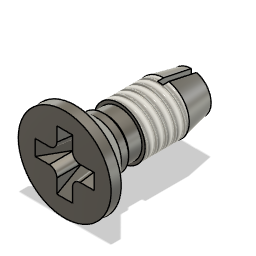
final_combined_updated (Autodesk Fusion 360 archive; units mm, degrees)
design "Type I Cross Recessed Flat Countersunk Head Tapping Screw ASME B18.6.5M M2.5x0.45 x 6 Type D Steel Grade 2 Plain"
description: Type I Cross Recessed Flat Countersunk Head Tapping Screw ASME B18.6.5M M2.5x0.45 x 6 Type D
part number: CRFCHTS ASME B18.6.5M - M2.5x0.45 x 6 - D - I Steel Grade 2 Plain
Autodesk Fusion 360 part; units mm, degrees
sketch "Sketch1" plane through (0, 0, 0) normal (0, 1, 0) x (1, 0, 0)
  line L0 (0, -2.68) -> (-2.2, -2.68)
  line L1 (-2.2, -2.68) -> (-2.2, -2.2)
  line L2 (-2.2, -2.2) -> (-1.18, -1.18)
  line L3 (-1.18, -1.18) -> (0, 0) construction
  line L4 (-1.25, 3.32) -> (0, 3.32)
  line L5 (0, 3.32) -> (0, -2.68)
  line L6 (-1.18, -1.18) -> (-1.18, -0.83)
  line L7 (-1.18, -0.83) -> (-1.0625, -0.7125)
  line L8 (-1.0625, -0.7125) -> (-1.0625, -0.08)
  line L9 (-1.0625, -0.08) -> (-1.25, -0.08)
  line L10 (-1.25, -0.08) -> (-1.25, 3.32)
  line L11 (-1.18, -1.18) -> (0, -1.18) construction
  dimension "d5" = 45
  dimension "d9" = 2.5
  dimension "d11" = 4.4
  dimension "d68" = 1.5
  dimension "d94" = 3.4
  dimension "d95" = 2.125
  dimension "d96" = 45
  dimension "d97" = 2.36
  dimension "d102" = 6
  dimension "d103" = 0.35
  constraint perpendicular L0 L1
  constraint collinear L2 L3
  constraint perpendicular L0 L5
  constraint collinear L3.end L0.start L4.end
  constraint coincident L3.end L5
  constraint coincident origin L3
  constraint horizontal L0
  constraint vertical L6
  constraint parallel L6 L8
  constraint perpendicular L8 L9
  constraint perpendicular L4 L10
  constraint vertical L10
  constraint coincident L5 L11.end
  constraint perpendicular L5 L11
  measures "d5" angle of L3 L5
  measures "d68" distance of L0 L2.end
  measures "d94" distance of L4 L9
  measures "d96" angle of L6 L7
  measures "d102" distance of L0.start L4
  measures "d103" distance of L6.end L11
revolve "Revolve1" add sketch "Sketch1" angle 360 about axis through (0, 0, -3.32) along (0, 0, 1) makes body 1
sketch "Sketch2" plane through (0, 0, 2.68) normal (0, 0, 1) x (1, 0, 0)
  line L0 (-0.37, 0.37) -> (-1.4, 0.37)
  line L1 (-1.4, 0.37) -> (-1.4, -0.37)
  line L2 (-1.4, -0.37) -> (-0.37, -0.37)
  line L3 (-0.37, -0.37) -> (-0.37, -1.4)
  line L4 (-0.37, -1.4) -> (0.37, -1.4)
  line L5 (0.37, -1.4) -> (0.37, -0.37)
  line L6 (0.37, -0.37) -> (1.4, -0.37)
  line L7 (1.4, -0.37) -> (1.4, 0.37)
  line L8 (1.4, 0.37) -> (0.37, 0.37)
  line L9 (0.37, 0.37) -> (0.37, 1.4)
  line L10 (0.37, 1.4) -> (-0.37, 1.4)
  line L11 (-0.37, 1.4) -> (-0.37, 0.37)
  dimension "d104" = 0.74
  dimension "d106" = 360
  dimension "d107" = 2.8
  constraint horizontal L0
  constraint perpendicular L0 L1
  constraint horizontal L2
  constraint vertical L0.start L2.end
  constraint coincident L0.start L11.end
  measures "d104" distance of L0 L1.end
  measures "d107" distance of L3.end L10
extrude "Extrude1" add sketch "Sketch2" against normal blind 1.78 draft -4 separate body makes body 2
draft "Draft1" angle -30 neutral plane through (0, 0, 2.68) pull (0, 0, 1) 4 faces at (1.3585, 0.0818, 2.0867) (-0.0818, 1.3585, 2.0867) (-0.0818, -1.3585, 2.0867) (-1.3585, 0.0818, 2.0867) on bodies 2
fillet "Fillet3" radius 0.364 4 edges at (0.3078, 0.3078, 1.79) (-0.3078, 0.3078, 1.79) (-0.3078, -0.3078, 1.79) (0.3078, -0.3078, 1.79) on bodies 2
combine "Combine1" operation cut target body 1 tool bodies 2
thread "Thread1" "ANSI Metric M Profile 2.5 M2.5x0.45 6g" major diameter 2.43 minor diameter 1.9165 pitch 0.45 angle 60 resizes the face on face at (-1.2484, 0.0623, -1.0533) on bodies 1
sketch "Sketch5" plane through (0, 0, 0) normal (0, 1, 0) x (1, 0, 0)
  line L0 (-1.275, 3.32) -> (-1.275, 1.72)
  line L1 (-1.275, 1.72) -> (-0.94, 3.32)
  line L2 (0, 3.32) -> (0, -2.68)
  line L3 (0, 3.32) -> (-1.275, 3.32)
  dimension "d81" = 1.275
  dimension "d110" = 0.94
  dimension "d111" = 1.6
  constraint vertical L0
  constraint coincident L2.start L3.start
  constraint perpendicular L0 L3
  constraint coincident L1.end L3
  measures "d81" distance of origin L0
  measures "d110" distance of L1.end L2
  measures "d111" distance of L0.end L3
revolve "Revolve2" cut sketch "Sketch5" angle 360 about axis through (0, 0, -3.32) along (0, 0, 1) bodies 1
sketch "Sketch6" plane through (0, 0, -3.32) normal (0, 0, -1) x (-1, 0, 0)
  line L0 (-0.25, 2.2) -> (0, 2.2)
  line L1 (0, 2.2) -> (0, 0)
  line L2 (0, 0) -> (-0.25, 0)
  circle A0 centre (0, 0) radius 0.94
  line L3 (-0.25, 2.2) -> (-0.25, 0)
  dimension "d112" = 0.25
  dimension "d113" = 2.2
  constraint horizontal L2
  constraint coincident L1.end L2.start
  constraint perpendicular L1 L2
  constraint perpendicular L0 L1
  constraint perpendicular L0 L3
  measures "d112" distance of L0.end L3
  measures "d113" distance of L1.end L0
extrude "Extrude2" cut sketch "Sketch6" against normal blind 1.6 contours L0 L1 A0 L3 | L1 L2 A0 L3 picked at (-0.1667, 0.302) bodies 1
equation "d5 = adsk_headang * 0.5"
equation "d9 = adsk_nomdia"
equation "d11 = adsk_headdia"
equation "adsk_nomlen = 6.00 mm"
equation "adsk_headh = 1.50 mm"
equation "adsk_headdia = 4.40 mm"
equation "adsk_nomdia = 2.50 mm"
equation "adsk_headang = 90.00 deg"
equation "adsk_phildia = 2.80 mm"
equation "d31 = -adsk_phildepth"
equation "adsk_philwidth = 0.74 mm"
equation "adsk_phildepth = 1.78 mm"
equation "adsk_startlen = 1.60 mm"
equation "d68 = adsk_headh"
equation "d73 = -adsk_startlen"
equation "adsk_endpointdia = 1.88 mm"
equation "d81 = adsk_nomdia * 0.51"
equation "d86 = ( adsk_nomdia * 0.5 ) * tan(90 deg - adsk_headang * 0.5) + adsk_headh"
equation "adsk_thrlen = 3.40 mm"
equation "adsk_grpdia = 2.36 mm"
equation "adsk_grplen = 0.35 mm"
equation "adsk_shlang = 45.00 deg"
equation "d94 = adsk_thrlen"
equation "d95 = adsk_shnkdia"
equation "d96 = adsk_shlang"
equation "d97 = adsk_grpdia"
equation "adsk_shnkdia = adsk_nomdia * 0.85"
equation "d102 = adsk_nomlen"
equation "d103 = adsk_grplen"
equation "d104 = adsk_philwidth"
equation "d107 = adsk_phildia"
equation "d109 = adsk_phildia * 0.13"
equation "d110 = adsk_endpointdia / 2"
equation "d111 = adsk_startlen"
equation "d112 = adsk_nomdia / 10"
equation "d113 = adsk_headdia / 2"

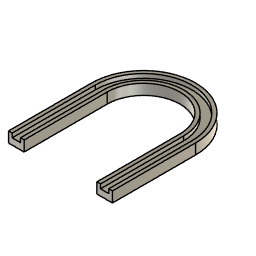
design "supporter"
Autodesk Fusion 360 part; units mm, degrees
sketch "Sketch1" plane through (0, 0, 0) normal (0, 0, 1) x (1, 0, 0)
  line L0 (-65, 0) -> (67.0686, 0)
  line L1 (-35, 0) -> (-35, -80)
  line L2 (-50, 0) -> (-50, -80)
  line L3 (35, 0) -> (35, -80)
  line L4 (50, 0) -> (50, -80)
  line L5 (35, -80) -> (50, -80)
  line L6 (-50, -80) -> (-35, -80)
  arc A0 (35, 0) -> (-35, 0) centre (0, 0) ccw
  arc A1 (50, 0) -> (-50, 0) centre (0, 0) ccw
  arc A2 (38.5, 0) -> (-38.5, 0) centre (0, 0) ccw
  arc A3 (46.5, 0) -> (-46.5, 0) centre (0, 0) ccw
  line L7 (-38.5, 0) -> (-38.5, -80)
  line L8 (-46.5, 0) -> (-46.5, -80)
  line L9 (38.5, 0) -> (38.5, -80)
  line L10 (46.5, 0) -> (46.5, -80)
  dimension "d1" = 70
  dimension "d2" = 100
  dimension "d3" = 80
  dimension "d4" = 80
  dimension "d5" = 80
  dimension "d8" = 77
  dimension "d9" = 93
  constraint coincident A0.centre A1.centre
  constraint horizontal L0
  constraint coincident L0 L1.start
  constraint tangent L1 A0
  constraint perpendicular L0 L1
  constraint coincident L0 L2.start
  constraint tangent L2 A1
  constraint coincident L0 L3.start
  constraint tangent L3 A0
  constraint coincident L0 L4.start
  constraint tangent L4 A1
  constraint perpendicular L4 L5
  constraint concentric A0 A3
  constraint coincident L0 A2.end
  constraint coincident L0 A2.start
  constraint coincident L0 A3.end
  constraint coincident L0 A3.start
  constraint coincident L6 L7.end
  constraint tangent A2 L7
  constraint coincident L6 L8.end
  constraint tangent A3 L8
  constraint coincident L5 L9.end
  constraint tangent A2 L9
  constraint coincident L5 L10.end
  constraint tangent A3 L10
  measures "d1" diameter of A0
  measures "d2" diameter of A1
  measures "d3" distance of L1.start L1.end
  measures "d4" distance of L2.start L2.end
  measures "d5" distance of L4.start L4.end
  measures "d8" diameter of A2
  measures "d9" diameter of A3
extrude "Extrude2" add sketch "Sketch1" along normal blind 6 contours L0 A1 A3 | L0 L2 L6 L8 | L0 L4 L5 L10 | L0 A0 A2 | L0 L1 L6 L7 | L0 L3 L5 L9 makes body 1 at (36.1667, -53.3333, 0) makes body 2 at (-47.6667, -53.3333, 0)
extrude "Extrude3" add sketch "Sketch1" along normal blind 2 separate body contours L0 A2 A3 | L0 L6 L7 L8 | L0 L5 L9 L10 makes body 3
extrude "Extrude4" add sketch "Sketch1" against normal blind 4.1 contours L0 A1 A3 | L0 L2 L6 L8 | L0 A2 A3 | L0 L6 L7 L8 | L0 L4 L5 L10 | L0 A0 A2 | L0 L1 L6 L7 | L0 L5 L9 L10 | L0 L3 L5 L9 bodies 1 2 3

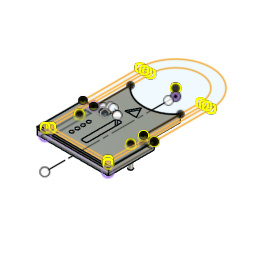
design "cap"
Autodesk Fusion 360 part; units mm, degrees
ref_plane "WorkPlane1" through (0, 0, 100) normal (0, 0, 1) x (1, 0, 0)
sketch "Sketch3" plane through (0, 0, 100) normal (0, 0, 1) x (1, 0, 0)
  line L0 (50, -80) -> (50, 0)
  arc A0 (50, 0) -> (-50, 0) centre (0, 0) ccw
  arc A1 (35, 0) -> (-35, 0) centre (0, 0) ccw
  line L1 (35, 0) -> (35, -80)
  line L2 (35, -80) -> (50, -80)
  line L3 (-50, 0) -> (-50, -80)
  line L4 (-50, -80) -> (-35, -80)
  line L5 (-35, -80) -> (-35, 0)
  circle A2 centre (-36, -99) radius 3
  circle A3 centre (36, -99) radius 3
  line L6 (40, -135) -> (-40, -135)
  line L7 (-40, -135) -> (-40, 0)
  line L8 (40, 0) -> (40, -135)
  line L9 (-44, -139) -> (-44, 0)
  line L10 (44, 0) -> (44, -139)
  line L11 (44, -139) -> (-44, -139)
  arc A4 (-35, -28.2843) -> (35, -28.2843) centre (0, 0) ccw
  line L12 (-35, -28.2843) -> (-35, -80)
  line L13 (-50, -80) -> (-50, -144)
  line L14 (-50, -144) -> (50, -144)
  line L15 (50, -144) -> (50, -80)
  line L16 (50, -80) -> (35, -80)
  line L17 (35, -28.2843) -> (35, -80)
  line L18 (-50, -80) -> (-35, -80)
  circle A5 centre (-36, -99) radius 2.8
  circle A6 centre (36, -99) radius 2.9
  dimension "d2" = 90
  dimension "d3" = 5.6
  dimension "d4" = 5.8
  dimension "d15" = 64
  constraint concentric A1 A4
  constraint coincident L5 A4.start
  constraint coincident L1 A4.end
  constraint coincident L4.end L5.start
  constraint coincident L3.end L4.start
  constraint perpendicular L11 L13
  constraint perpendicular L10 L14
  constraint coincident L0.start L2.end
  constraint perpendicular L14 L15
  constraint coincident L1.end L2.start
  constraint concentric A2 A5
  constraint concentric A3 A6
  measures "d2" diameter of A4
  measures "d3" diameter of A5
  measures "d4" diameter of A6
  measures "d15" distance of L14.end L0.start
extrude "Extrude1" add sketch "Sketch3" against normal blind 10 contours L2 L4 L9 L10 L11 L13 L14 L15 L16 L18 | L2 L4 L6 L7 L8 L9 L10 L11 L16 L18 | L1 L2 L4 L5 L6 L7 L8 A4 L12 L16 L17 L18 makes body 1
extrude "Extrude2" add sketch "Sketch3" against normal blind 30 separate body contours A5 | A6 makes body 2 at (-33.541, -100.3391, 80) makes body 3 at (37.1927, -96.3566, 80)
sketch "Sketch6" plane through (0, 0, 90) normal (0, 0, -1) x (1, 0, 0)
  circle A0 centre (36, 99) radius 3
  circle A1 centre (-36, 99) radius 3
  line L0 (50, 144) -> (-50, 144)
  line L1 (-50, 144) -> (-50, 80)
  line L2 (-50, 80) -> (-35, 80)
  line L3 (-35, 80) -> (-35, 28.2843)
  arc A2 (35, 28.2843) -> (-35, 28.2843) centre (0, 0) ccw
  line L4 (35, 28.2843) -> (35, 80)
  line L5 (35, 80) -> (50, 80)
  line L6 (50, 80) -> (50, 144)
  line L7 (35, 80) -> (42.5, 80)
  line L8 (42.5, 80) -> (46.5, 80)
  line L9 (42.5, 80) -> (39, 80)
  line L10 (46.5, 80) -> (46.5, 133)
  line L11 (39, 80) -> (39, 132)
  line L12 (0, 0) -> (0, 10)
  line L13 (0, 10) -> (0, 183.5284)
  line L14 (0, 10) -> (0, 183.5284)
  line L15 (-39, 80) -> (-39, 132)
  line L16 (-46.5, 80) -> (-46.5, 133)
  line L17 (-42.5, 80) -> (-39, 80)
  line L18 (-42.5, 80) -> (-46.5, 80)
  line L19 (-39, 132) -> (39, 132)
  line L20 (46.5, 133) -> (46.5, 142)
  line L21 (-46.5, 133) -> (-46.5, 142)
  line L22 (-46.5, 142) -> (46.5, 142)
  line L23 (44, 139) -> (-44, 139)
  dimension "d9" = 4
  dimension "d10" = 3.5
  dimension "d11" = 53
  dimension "d12" = 52
  dimension "d19" = 3
  constraint coincident L4.end L5.start
  constraint midpoint L5 L7.end
  constraint parallel L5 L8
  constraint parallel L7 L9
  constraint perpendicular L8 L10
  constraint perpendicular L9 L11
  constraint coincident A2.centre L12.start
  constraint vertical L12
  constraint parallel L12 L13
  constraint symmetric L7.end L13 L17.start
  constraint symmetric L8.end L13 L16.start
  constraint symmetric L9.end L13 L15.start
  constraint symmetric L10.end L13 L16.end
  constraint symmetric L11.end L13 L15.end
  constraint symmetric L12.end L13 L14.start
  constraint symmetric L14.end L13 L13.end
  constraint parallel L10 L20
  constraint parallel L16 L21
  constraint perpendicular L20 L22
  measures "d9" distance of L7.end L8.end
  measures "d10" distance of L7.end L9.end
  measures "d11" distance of L8.end L10.end
  measures "d12" distance of L9.end L11.end
  measures "d19" distance of L22 L23
extrude "Extrude4" cut sketch "Sketch6" against normal blind 4 contours L5 L7 L8 L9 L10 L11 L13 L14 L19 L20 L22 | L2 L13 L14 L15 L16 L17 L18 L19 L21 L22 bodies 1
sketch "Sketch7" plane through (0, 0, 100) normal (0, 0, 1) x (1, 0, 0)
  line L0 (-20, -101.7213) -> (-20, -125.7213)
  circle A0 centre (-20, -101.7213) radius 2.5
  circle A1 centre (-20, -125.7213) radius 2.5
  circle A2 centre (-20, -117.7213) radius 2.5
  circle A3 centre (-20, -109.7213) radius 2.5
  dimension "d20" = 5
  dimension "d21" = 24
  dimension "d22" = 5
  dimension "d23" = 5
  dimension "d24" = 5
  dimension "d28" = 8
  dimension "d30" = 8
  dimension "d31" = 8
  constraint vertical L0
  constraint coincident L0.start A0.centre
  constraint coincident L0.end A1.centre
  constraint coincident L0 A2.centre
  constraint coincident L0 A3.centre
  measures "d20" diameter of A0
  measures "d21" distance of L0.start L0.end
  measures "d22" diameter of A1
  measures "d23" diameter of A2
  measures "d24" diameter of A3
  measures "d28" distance of L0.start A3.centre
  measures "d30" distance of A2.centre A3.centre
  measures "d31" distance of L0.end A2.centre
extrude "Extrude5" cut sketch "Sketch7" against normal blind 45 bodies 1
sketch "Sketch8" plane through (0, 0, 100) normal (0, 0, 1) x (1, 0, 0)
  line L0 (-27, -68.082) -> (-14.9, -68.082)
  line L1 (-14.9, -68.082) -> (-14.9, -80.182)
  line L2 (-14.9, -80.182) -> (-27, -80.182)
  line L3 (-27, -80.182) -> (-27, -68.082)
  line L4 (-27, -80.182) -> (-23, -80.182)
  circle A0 centre (-23, -80.182) radius 1
  line L5 (-23, -80.182) -> (-19, -80.182)
  circle A1 centre (-19, -80.182) radius 1
  line L6 (-27, -68.082) -> (-27, -74.082)
  line L7 (-27, -74.082) -> (-7.7924, -74.082)
  line L8 (-27, -74.082) -> (-7.7924, -74.082)
  circle A2 centre (-23, -67.982) radius 1
  circle A3 centre (-19, -67.982) radius 1
  point P0 (-35, -80)
  dimension "d34" = 12.1
  dimension "d35" = 12.1
  dimension "d36" = 4
  dimension "d37" = 2
  dimension "d38" = 4
  dimension "d39" = 2
  dimension "d40" = 6
  dimension "d41" = 8
  constraint horizontal L0
  constraint vertical L1
  constraint horizontal L2
  constraint vertical L3
  constraint perpendicular L3 L4
  constraint coincident L4.end A0.centre
  constraint parallel L2 L5
  constraint coincident L5.end A1.centre
  constraint perpendicular L0 L6
  constraint perpendicular L1 L7
  constraint symmetric A0 L7 A2
  constraint symmetric A1 L7 A3
  constraint symmetric L6.end L7 L8.start
  constraint symmetric L8.end L7 L7.end
  measures "d34" distance of L0.start L0.end
  measures "d35" distance of L0.start L2.end
  measures "d36" distance of L2.end L4.end
  measures "d37" diameter of A0
  measures "d38" distance of L4.end L5.end
  measures "d39" diameter of A1
  measures "d40" distance of L0.start L6.end
  measures "d41" horizontal distance of L2.end P0
extrude "Extrude6" cut sketch "Sketch8" against normal blind 17 contours L0 A2 | L0 A2 | L0 A3 | L0 A3 | L2 L4 A0 L5 | L2 L4 A0 L5 | L2 L5 A1 | L2 L5 A1 bodies 1
extrude "Extrude7" cut sketch "Sketch8" against normal blind 7 contours L0 L1 L3 L6 L7 L8 A2 A3 | L1 L2 L3 L4 A0 L5 A1 L7 L8 bodies 1
sketch "Sketch9" plane through (0, 0, 100) normal (0, 0, 1) x (1, 0, 0)
  line L0 (4, -79) -> (-4, -79)
  line L1 (-4, -79) -> (-4, -129)
  line L2 (-4, -129) -> (4, -129)
  line L3 (4, -129) -> (4, -79)
  line L4 (4, -79) -> (-4, -129) construction
  line L5 (-4, -79) -> (4, -129) construction
  line L6 (-50, -144) -> (50, -144)
  point P0 (0, -104)
  dimension "d46" = 8
  dimension "d47" = 50
  dimension "d48" = 15
  constraint horizontal L0
  constraint perpendicular L0 L1
  constraint parallel L0 L2
  constraint parallel L1 L3
  constraint coincident L4 P0
  constraint coincident L5 P0
  measures "d46" distance of L1.end L2.end
  measures "d47" distance of L0.end L1.end
  measures "d48" distance of L2 L6
extrude "Extrude8" cut sketch "Sketch9" against normal blind 55 bodies 1
fillet "Fillet1" radius 1.5 4 edges at (-4, -79, 95) (4, -79, 95) (-4, -129, 95) (4, -129, 95) on bodies 1
fillet "Fillet2" radius 3 1 edges at (0, -144, 100) on bodies 1
sketch "Sketch12" plane through (0, 0, 100) normal (0, 0, 1) x (1, 0, 0)
  line L0 (0, -63) -> (8, -63)
  line L1 (0, -63) -> (-8, -63)
  line L2 (-8, -63) -> (-0.019, -47.9899)
  line L3 (-8, -63) -> (4.6601, -63) construction
  line L4 (0, -10) -> (0, -183.5284)
  line L5 (-0.019, -47.9899) -> (7.962, -63)
  line L6 (-0.019, -47.9899) -> (16.981, -47.9899) construction
  dimension "d78" = 8
  dimension "d79" = 8
  dimension "d80" = 17
  dimension "d81" = 62
  dimension "d82" = 17
  dimension "d83" = 62
  constraint horizontal L0
  constraint parallel L0 L1
  constraint horizontal L3
  constraint coincident L0.start L4
  constraint horizontal L6
  measures "d78" distance of L0.start L0.end
  measures "d79" distance of L0.start L1.end
  measures "d80" distance of L1.end L2.end
  measures "d81" angle of L2 L3
  measures "d82" distance of L2.end L5.end
  measures "d83" angle of L5 L6
extrude "Extrude10" cut sketch "Sketch12" against normal blind 2 bodies 1
equation "d7 = -23 mm - 7 mm"
